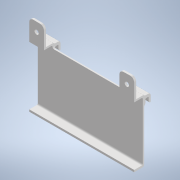
# Autodesk Inventor part: akkum_cup
Saved by Autodesk Inventor 2022 (Build 260153000, 153)
## iProperties
Created: 2024-11-13
Part Number: akkum_cup
Material: Типовые
Document SubType Name: Modeling
Designer: Andrey
Density: 1 g/cm^3
Appearance: По умолчанию
Author: Andrey
Autodesk Inventor part; units mm, degrees
ref_plane "YZ Plane" through (0, 0, 0) normal (1, 0, 0) x (0, 1, 0)
sketch "Эскиз1" plane through (0, 0, 0) normal (0, 0, 1) x (1, 0, 0)
  line L0 (39.5, 4.130031) -> (39.5, 47.075)
  line L1 (17.068713, 47.075) -> (39.5, 47.075)
  line L2 (17.068713, 47.075) -> (17.068713, 32.075)
  line L3 (17.068713, 32.075) -> (19.451364, 32.075)
  line L4 (19.451364, 32.075) -> (19.451364, 22.075)
  line L5 (19.451364, 22.075) -> (17.068713, 22.075)
  line L6 (17.068713, 22.075) -> (17.068713, 21.075)
  line L7 (17.068713, 21.075) -> (-5.922093, 21.075)
  line L8 (-5.922093, 21.075) -> (-5.922093, 47.075)
  line L9 (-39.5, 47.075) -> (-5.922093, 47.075)
  line L10 (-39.5, 47.075) -> (-39.5, 4.130031)
  line L11 (-39.5, 4.130031) -> (-43.5, 4.130031)
  line L12 (-43.5, -51.925) -> (-43.5, 4.130031)
  line L13 (43.5, -51.925) -> (-43.5, -51.925)
  line L14 (43.5, 4.130031) -> (43.5, -51.925)
  line L15 (43.5, 4.130031) -> (39.5, 4.130031)
  line L16 (-40, 47.075) -> (40, 47.075)
  line L17 (40, 47.075) -> (40, 7.075)
  line L18 (40, 7.075) -> (-40, 7.075)
  line L19 (-40, 7.075) -> (-40, 47.075)
  line L20 (39.5, -51.925) -> (-39.5, -51.925)
  line L21 (-39.5, -51.925) -> (-39.5, 106.075)
  line L22 (-39.5, 106.075) -> (39.5, 106.075)
  line L23 (39.5, 106.075) -> (39.5, -51.925)
  line L24 (-40, 50.145438) -> (-43.5, 50.145438)
  line L25 (-43.5, 50.145438) -> (-43.5, 87.075)
  line L26 (-43.5, 87.075) -> (-62.794737, 87.075)
  line L27 (-62.794737, 87.075) -> (-62.794737, -32.925)
  line L28 (-62.794737, -32.925) -> (-43.5, -32.925)
  line L29 (-43.5, -32.925) -> (-43.5, 5.130031)
  line L30 (-43.5, 5.130031) -> (43.5, 5.130031)
  line L31 (43.5, 5.130031) -> (43.5, -32.925)
  line L32 (43.5, -32.925) -> (62.794737, -32.925)
  line L33 (62.794737, -32.925) -> (62.794737, 87.075)
  line L34 (62.794737, 87.075) -> (43.5, 87.075)
  line L35 (43.5, 87.075) -> (43.5, 50.145438)
  line L36 (43.5, 50.145438) -> (40, 50.145438)
  line L37 (40, 50.145438) -> (40, 49.145438)
  line L38 (40, 49.145438) -> (27.613813, 49.145438)
  line L39 (27.613813, 49.145438) -> (27.613813, 50.271275)
  line L40 (27.613813, 50.271275) -> (10.238021, 50.271275)
  line L41 (10.238021, 50.271275) -> (10.238021, 49.145438)
  line L42 (10.238021, 49.145438) -> (5, 49.145438)
  line L43 (5, 49.145438) -> (5, 52.145438)
  line L44 (5, 52.145438) -> (-5, 52.145438)
  line L45 (-5, 52.145438) -> (-5, 49.145438)
  line L46 (-5, 49.145438) -> (-10.238021, 49.145438)
  line L47 (-10.238021, 49.145438) -> (-10.238021, 50.271275)
  line L48 (-10.238021, 50.271275) -> (-27.613813, 50.271275)
  line L49 (-27.613813, 50.271275) -> (-27.613813, 49.145438)
  line L50 (-27.613813, 49.145438) -> (-40, 49.145438)
  line L51 (-40, 49.145438) -> (-40, 50.145438)
  line L52 (-40.5, -9.071748) -> (-40.5, -29.675)
  line L53 (-40.5, -29.675) -> (-25.5, -29.675)
  line L54 (-25.5, -29.675) -> (-25.5, -9.071748)
  line L55 (-25.5, -9.071748) -> (-40.5, -9.071748)
  circle A0 centre (-35.935126, 58.395438) radius 2.1
  circle A1 centre (-23.0037, 78.773688) radius 2.1
  circle A2 centre (23.0037, 78.773688) radius 2.1
  circle A3 centre (35.954001, 58.395438) radius 2.1
  line L56 (-5, 87.075) -> (5, 87.075)
  line L57 (5, 87.075) -> (5, 106.075)
  line L58 (5, 106.075) -> (52.763624, 106.075)
  spline S0 degree 4 poles (64.11012, 98.855268) (61.979597, 102.169879) (57.930304, 105.392192) (55.716138, 106.075) (52.763624, 106.075) knots 0 0 0 0 0 1 1 1 1 1
  spline S1 degree 2 poles (66.794737, 82.075) (67.198697, 94.050143) (64.11012, 98.855268) knots 0 0 0 0.59571899 0.59571899 0.59571899
  line L59 (66.794737, -27.925) -> (66.794737, 82.075)
  spline S2 degree 2 poles (66.794737, -27.925) (67.198697, -39.900143) (64.11012, -44.705268) knots 0 0 0 0.59571899 0.59571899 0.59571899
  spline S3 degree 4 poles (64.11012, -44.705268) (64.099074, -44.722454) (64.087976, -44.739637) (64.076827, -44.756817) (64.065627, -44.773995) knots 0 0 0 0 0 1 1 1 1 1
  spline S4 degree 4 poles (63.235072, -45.91909) (63.456659, -45.667632) (63.669141, -45.393003) (63.87219, -45.095007) (64.065627, -44.773995) knots 0 0 0 0 0 1 1 1 1 1
  spline S5 degree 4 poles (63.235072, -45.91909) (60.901345, -48.850089) (57.514512, -51.362629) (55.443125, -51.925) (52.763624, -51.925) knots 0.09246802 0.09246802 0.09246802 0.09246802 0.09246802 1 1 1 1 1
  line L60 (6, -51.925) -> (52.763624, -51.925)
  line L61 (6, -51.925) -> (6, -36.071748)
  arc A4 (6, -36.071748) -> (5, -35.071748) centre (5, -36.071748) ccw
  line L62 (5, -35.071748) -> (-5, -35.071748)
  arc A5 (-5, -35.071748) -> (-6, -36.071748) centre (-5, -36.071748) ccw
  line L63 (-6, -36.071748) -> (-6, -51.925)
  line L64 (-52.763624, -51.925) -> (-6, -51.925)
  spline S6 degree 4 poles (-64.11012, -44.705268) (-61.979597, -48.019879) (-57.930304, -51.242192) (-55.716138, -51.925) (-52.763624, -51.925) knots 0 0 0 0 0 1 1 1 1 1
  spline S7 degree 2 poles (-66.794737, -27.925) (-67.198697, -39.900143) (-64.11012, -44.705268) knots 0 0 0 0.59571899 0.59571899 0.59571899
  line L65 (-66.794737, 82.075) -> (-66.794737, -27.925)
  spline S8 degree 2 poles (-64.11012, 98.855268) (-67.198697, 94.050143) (-66.794737, 82.075) knots -0.59571899 -0.59571899 -0.59571899 0 0 0
  spline S9 degree 4 poles (-64.11012, 98.855268) (-61.979597, 102.169879) (-57.930304, 105.392192) (-55.716138, 106.075) (-52.763624, 106.075) knots 0 0 0 0 0 1 1 1 1 1
  line L66 (-52.763624, 106.075) -> (-5, 106.075)
  line L67 (-5, 106.075) -> (-5, 87.075)
  line L68 (-33.1, -33.525) -> (-40.1, -33.525)
  line L69 (-40.1, -33.525) -> (-40.1, -47.625)
  line L70 (-40.1, -47.625) -> (-33.1, -47.625)
  line L71 (-33.1, -47.625) -> (-33.1, -33.525)
  line L72 (40.1, -33.675) -> (33.1, -33.675)
  line L73 (33.1, -33.675) -> (33.1, -47.625)
  line L74 (33.1, -47.625) -> (40.1, -47.625)
  line L75 (40.1, -47.625) -> (40.1, -33.675)
  line L76 (3.8, 77.044784) -> (-15.7, 77.044784)
  arc A6 (-15.7, 77.044784) -> (-18.7, 74.044784) centre (-15.7, 74.044784) ccw
  line L77 (-18.7, 74.044784) -> (-18.7, 60.781085)
  arc A7 (-18.7, 60.781085) -> (-15.7, 57.781085) centre (-15.7, 60.781085) ccw
  line L78 (-15.7, 57.781085) -> (3.8, 57.781085)
  arc A8 (3.8, 57.781085) -> (6.8, 60.781085) centre (3.8, 60.781085) ccw
  line L79 (6.8, 60.781085) -> (6.8, 74.044784)
  arc A9 (6.8, 74.044784) -> (3.8, 77.044784) centre (3.8, 74.044784) ccw
  line L80 (39.5, 49.145438) -> (-39.5, 49.145438)
  line L81 (-37.533703, 49.795438) -> (-66.794737, 49.795438)
  line L82 (-66.794737, 49.795438) -> (66.794737, 49.795438)
  line L83 (66.794737, 3.630031) -> (-65.776453, 3.630031)
  line L84 (-40, 50.145438) -> (-43.5, 50.145438)
  line L85 (-43.5, 50.145438) -> (-43.5, 87.075)
  line L86 (-43.5, 87.075) -> (-62.794737, 87.075)
  line L87 (-62.794737, 87.075) -> (-62.794737, -32.925)
  line L88 (-62.794737, -32.925) -> (-43.5, -32.925)
  line L89 (-43.5, -32.925) -> (-43.5, 5.130031)
  line L90 (-43.5, 5.130031) -> (43.5, 5.130031)
  line L91 (43.5, 5.130031) -> (43.5, -32.925)
  line L92 (43.5, -32.925) -> (62.794737, -32.925)
  line L93 (62.794737, -32.925) -> (62.794737, 87.075)
  line L94 (62.794737, 87.075) -> (43.5, 87.075)
  line L95 (43.5, 87.075) -> (43.5, 50.145438)
  line L96 (43.5, 50.145438) -> (40, 50.145438)
  line L97 (40, 50.145438) -> (40, 49.145438)
  line L98 (40, 49.145438) -> (27.613813, 49.145438)
  line L99 (27.613813, 49.145438) -> (27.613813, 50.271275)
  line L100 (27.613813, 50.271275) -> (10.238021, 50.271275)
  line L101 (10.238021, 50.271275) -> (10.238021, 49.145438)
  line L102 (10.238021, 49.145438) -> (5, 49.145438)
  line L103 (5, 49.145438) -> (5, 52.145438)
  line L104 (5, 52.145438) -> (-5, 52.145438)
  line L105 (-5, 52.145438) -> (-5, 49.145438)
  line L106 (-5, 49.145438) -> (-10.238021, 49.145438)
  line L107 (-10.238021, 49.145438) -> (-10.238021, 50.271275)
  line L108 (-10.238021, 50.271275) -> (-27.613813, 50.271275)
  line L109 (-27.613813, 50.271275) -> (-27.613813, 49.145438)
  line L110 (-27.613813, 49.145438) -> (-40, 49.145438)
  line L111 (-40, 49.145438) -> (-40, 50.145438)
  line L112 (-40.5, -9.071748) -> (-40.5, -29.675)
  line L113 (-40.5, -29.675) -> (-25.5, -29.675)
  line L114 (-25.5, -29.675) -> (-25.5, -9.071748)
  line L115 (-25.5, -9.071748) -> (-40.5, -9.071748)
  circle A10 centre (-35.935126, 58.395438) radius 2.1
  circle A11 centre (-23.0037, 78.773688) radius 2.1
  circle A12 centre (23.0037, 78.773688) radius 2.1
  circle A13 centre (35.954001, 58.395438) radius 2.1
  line L116 (-5, 87.075) -> (5, 87.075)
  line L117 (5, 87.075) -> (5, 106.075)
  line L118 (5, 106.075) -> (52.763624, 106.075)
  spline S10 degree 4 poles (64.11012, 98.855268) (61.979597, 102.169879) (57.930304, 105.392192) (55.716138, 106.075) (52.763624, 106.075) knots 0 0 0 0 0 1 1 1 1 1
  spline S11 degree 2 poles (66.794737, 82.075) (67.198697, 94.050143) (64.11012, 98.855268) knots 0 0 0 0.59571899 0.59571899 0.59571899
  line L119 (66.794737, -27.925) -> (66.794737, 82.075)
  spline S12 degree 2 poles (66.794737, -27.925) (67.198697, -39.900143) (64.11012, -44.705268) knots 0 0 0 0.59571899 0.59571899 0.59571899
  spline S13 degree 4 poles (64.11012, -44.705268) (64.099074, -44.722454) (64.087976, -44.739637) (64.076827, -44.756817) (64.065627, -44.773995) knots 0 0 0 0 0 1 1 1 1 1
  spline S14 degree 4 poles (63.235072, -45.91909) (63.456659, -45.667632) (63.669141, -45.393003) (63.87219, -45.095007) (64.065627, -44.773995) knots 0 0 0 0 0 1 1 1 1 1
  spline S15 degree 4 poles (63.235072, -45.91909) (60.901345, -48.850089) (57.514512, -51.362629) (55.443125, -51.925) (52.763624, -51.925) knots 0.09246802 0.09246802 0.09246802 0.09246802 0.09246802 1 1 1 1 1
  line L120 (6, -51.925) -> (52.763624, -51.925)
  line L121 (6, -51.925) -> (6, -36.071748)
  arc A14 (6, -36.071748) -> (5, -35.071748) centre (5, -36.071748) ccw
  line L122 (5, -35.071748) -> (-5, -35.071748)
  arc A15 (-5, -35.071748) -> (-6, -36.071748) centre (-5, -36.071748) ccw
  line L123 (-6, -36.071748) -> (-6, -51.925)
  line L124 (-52.763624, -51.925) -> (-6, -51.925)
  spline S16 degree 4 poles (-64.11012, -44.705268) (-61.979597, -48.019879) (-57.930304, -51.242192) (-55.716138, -51.925) (-52.763624, -51.925) knots 0 0 0 0 0 1 1 1 1 1
  spline S17 degree 2 poles (-66.794737, -27.925) (-67.198697, -39.900143) (-64.11012, -44.705268) knots 0 0 0 0.59571899 0.59571899 0.59571899
  line L125 (-66.794737, 82.075) -> (-66.794737, -27.925)
  spline S18 degree 2 poles (-64.11012, 98.855268) (-67.198697, 94.050143) (-66.794737, 82.075) knots -0.59571899 -0.59571899 -0.59571899 0 0 0
  spline S19 degree 4 poles (-64.11012, 98.855268) (-61.979597, 102.169879) (-57.930304, 105.392192) (-55.716138, 106.075) (-52.763624, 106.075) knots 0 0 0 0 0 1 1 1 1 1
  line L126 (-52.763624, 106.075) -> (-5, 106.075)
  line L127 (-5, 106.075) -> (-5, 87.075)
  line L128 (-33.1, -33.525) -> (-40.1, -33.525)
  line L129 (-40.1, -33.525) -> (-40.1, -47.625)
  line L130 (-40.1, -47.625) -> (-33.1, -47.625)
  line L131 (-33.1, -47.625) -> (-33.1, -33.525)
  line L132 (40.1, -33.675) -> (33.1, -33.675)
  line L133 (33.1, -33.675) -> (33.1, -47.625)
  line L134 (33.1, -47.625) -> (40.1, -47.625)
  line L135 (40.1, -47.625) -> (40.1, -33.675)
  line L136 (3.8, 77.044784) -> (-15.7, 77.044784)
  arc A16 (-15.7, 77.044784) -> (-18.7, 74.044784) centre (-15.7, 74.044784) ccw
  line L137 (-18.7, 74.044784) -> (-18.7, 60.781085)
  arc A17 (-18.7, 60.781085) -> (-15.7, 57.781085) centre (-15.7, 60.781085) ccw
  line L138 (-15.7, 57.781085) -> (3.8, 57.781085)
  arc A18 (3.8, 57.781085) -> (6.8, 60.781085) centre (3.8, 60.781085) ccw
  line L139 (6.8, 60.781085) -> (6.8, 74.044784)
  arc A19 (6.8, 74.044784) -> (3.8, 77.044784) centre (3.8, 74.044784) ccw
  line L140 (27.613813, 49.145438) -> (27.613813, 47.075)
  line L141 (-27.613813, 49.145438) -> (-27.613813, 47.075)
  line L142 (-28.408002, 50.795438) -> (-28.408002, 49.795438)
  line L143 (28.408002, 49.795438) -> (28.408002, 50.795438)
  line L144 (28.408002, 50.795438) -> (43.5, 50.795438)
  line L145 (-43.5, 50.795438) -> (-28.408002, 50.795438)
  line L146 (43.5, 50.795438) -> (-43.5, 50.795438)
  line L147 (43.5, 50.495438) -> (-43.5, 50.495438)
  line L148 (-28.408002, 50.495438) -> (-28.408002, 47.075)
  line L149 (28.408002, 50.495438) -> (28.408002, 47.075)
  point P0 (0, 0)
  point P1 (39.5, 49.795438)
  point P2 (27.613813, 49.795438)
  point P3 (-27.613813, 49.795438)
  point P4 (-39.5, 49.795438)
  point P5 (-39.5, 3.630031)
  point P6 (39.5, 3.630031)
  point P7 (-39.5, 50.495438)
  point P8 (39.5, 50.495438)
  dimension "d0" = 1.5
  dimension "d7" = 0.3
  constraints: 32 end point, 13 point on line, 7 perpendicular, 4 collinear, 4 parallel, 3 horizontal, 2 vertical, 6 other
  measures "d0" distance between parallel lines of L30 L83
  measures "d7" distance between parallel lines of L146 L147
extrude "Выдавливание1" add sketch "Эскиз1" along normal blind 2 contours L23 L83 L21 L10 L30 L0 | L30 L10 L18 L0 | L18 L10 L9 L8 L7 L6 L5 L4 L3 L2 L1 L0 | L1 L149 L38 L23 | L38 L149 L82 L23 | L21 L50 L148 L9 | L82 L143 L147 L23 | L21 L81 L82 L148 L50 | L2 L3 L4 L5 L6 L7 L8 L16 | L21 L147 L142 L82 L81
sketch "Эскиз2" plane through (-39.5, 3.630031, 0) normal (-1, 0, 0) x (0, 0, 1)
  line L0 (0, 0) -> (2, 0)
  line L1 (1, 0) -> (1, 46.165408)
  line L2 (0, 46.165408) -> (2, 46.165408)
  line L3 (0, 46.865408) -> (0, 0)
  line L4 (0, 0) -> (2, 0)
  line L5 (2, 46.865408) -> (2, 0)
  line L6 (0, 46.865408) -> (2, 46.865408)
  line L7 (0, 46.865408) -> (2, 46.865408)
  line L8 (1, 46.865408) -> (1, 0)
  point P0 (0, -3.630031)
  point P1 (0, 0)
  constraints: 4 end point, 3 midpoint, 1 collinear
extrude "Выдавливание2" cut sketch "Эскиз2" against normal up to surface (79 mm away) contours L3 L2 L1 L0 | L3 L6 L8 L2
ref_plane "РабПлоскость1" through (-67.197727, -51.925, 8.5) normal (0, 0, -1) x (0, 1, 0)
sketch "Эскиз3" plane through (0, 0, 2) normal (0, 0, 1) x (1, 0, 0)
  line L0 (39.5, 3.630031) -> (39.5, 50.495438)
  line L1 (-39.5, 50.495438) -> (-39.5, 3.630031)
  line L2 (-39.5, 3.630031) -> (39.5, 3.630031)
  line L3 (-27.613813, 49.795438) -> (-39.5, 49.795438)
  line L4 (39.5, 3.630031) -> (39.5, 50.495438)
  line L5 (-39.5, 49.795438) -> (39.5, 49.795438)
  line L6 (39.5, 49.795438) -> (39.5, 49.145438)
  line L7 (39.5, 49.145438) -> (-39.5, 49.145438)
  line L8 (-39.5, 49.145438) -> (-39.5, 49.795438)
  line L9 (-40, 50.145438) -> (-43.5, 50.145438)
  line L10 (-43.5, 50.145438) -> (-43.5, 87.075)
  line L11 (-43.5, 87.075) -> (-62.794737, 87.075)
  line L12 (-62.794737, 87.075) -> (-62.794737, -32.925)
  line L13 (-62.794737, -32.925) -> (-43.5, -32.925)
  line L14 (-43.5, -32.925) -> (-43.5, 5.130031)
  line L15 (-43.5, 5.130031) -> (43.5, 5.130031)
  line L16 (43.5, 5.130031) -> (43.5, -32.925)
  line L17 (43.5, -32.925) -> (62.794737, -32.925)
  line L18 (62.794737, -32.925) -> (62.794737, 87.075)
  line L19 (62.794737, 87.075) -> (43.5, 87.075)
  line L20 (43.5, 87.075) -> (43.5, 50.145438)
  line L21 (43.5, 50.145438) -> (40, 50.145438)
  line L22 (40, 50.145438) -> (40, 49.145438)
  line L23 (40, 49.145438) -> (27.613813, 49.145438)
  line L24 (27.613813, 49.145438) -> (27.613813, 50.271275)
  line L25 (27.613813, 50.271275) -> (10.238021, 50.271275)
  line L26 (10.238021, 50.271275) -> (10.238021, 49.145438)
  line L27 (10.238021, 49.145438) -> (5, 49.145438)
  line L28 (5, 49.145438) -> (5, 52.145438)
  line L29 (5, 52.145438) -> (-5, 52.145438)
  line L30 (-5, 52.145438) -> (-5, 49.145438)
  line L31 (-5, 49.145438) -> (-10.238021, 49.145438)
  line L32 (-10.238021, 49.145438) -> (-10.238021, 50.271275)
  line L33 (-10.238021, 50.271275) -> (-27.613813, 50.271275)
  line L34 (-27.613813, 50.271275) -> (-27.613813, 49.145438)
  line L35 (-27.613813, 49.145438) -> (-40, 49.145438)
  line L36 (-40, 49.145438) -> (-40, 50.145438)
  line L37 (-40.5, -9.071748) -> (-40.5, -29.675)
  line L38 (-40.5, -29.675) -> (-25.5, -29.675)
  line L39 (-25.5, -29.675) -> (-25.5, -9.071748)
  line L40 (-25.5, -9.071748) -> (-40.5, -9.071748)
  circle A0 centre (-35.935126, 58.395438) radius 2.1
  circle A1 centre (-23.0037, 78.773688) radius 2.1
  circle A2 centre (23.0037, 78.773688) radius 2.1
  circle A3 centre (35.954001, 58.395438) radius 2.1
  line L41 (-5, 87.075) -> (5, 87.075)
  line L42 (5, 87.075) -> (5, 106.075)
  line L43 (5, 106.075) -> (52.763624, 106.075)
  spline S0 degree 4 poles (64.11012, 98.855268) (61.979597, 102.169879) (57.930304, 105.392192) (55.716138, 106.075) (52.763624, 106.075) knots 0 0 0 0 0 1 1 1 1 1
  spline S1 degree 2 poles (66.794737, 82.075) (67.198697, 94.050143) (64.11012, 98.855268) knots 0 0 0 0.59571899 0.59571899 0.59571899
  line L44 (66.794737, -27.925) -> (66.794737, 82.075)
  spline S2 degree 2 poles (66.794737, -27.925) (67.198697, -39.900143) (64.11012, -44.705268) knots 0 0 0 0.59571899 0.59571899 0.59571899
  spline S3 degree 4 poles (64.11012, -44.705268) (64.099074, -44.722454) (64.087976, -44.739637) (64.076827, -44.756817) (64.065627, -44.773995) knots 0 0 0 0 0 1 1 1 1 1
  spline S4 degree 4 poles (63.235072, -45.91909) (63.456659, -45.667632) (63.669141, -45.393003) (63.87219, -45.095007) (64.065627, -44.773995) knots 0 0 0 0 0 1 1 1 1 1
  spline S5 degree 4 poles (63.235072, -45.91909) (60.901345, -48.850089) (57.514512, -51.362629) (55.443125, -51.925) (52.763624, -51.925) knots 0.09246802 0.09246802 0.09246802 0.09246802 0.09246802 1 1 1 1 1
  line L45 (6, -51.925) -> (52.763624, -51.925)
  line L46 (6, -51.925) -> (6, -36.071748)
  arc A4 (6, -36.071748) -> (5, -35.071748) centre (5, -36.071748) ccw
  line L47 (5, -35.071748) -> (-5, -35.071748)
  arc A5 (-5, -35.071748) -> (-6, -36.071748) centre (-5, -36.071748) ccw
  line L48 (-6, -36.071748) -> (-6, -51.925)
  line L49 (-52.763624, -51.925) -> (-6, -51.925)
  spline S6 degree 4 poles (-64.11012, -44.705268) (-61.979597, -48.019879) (-57.930304, -51.242192) (-55.716138, -51.925) (-52.763624, -51.925) knots 0 0 0 0 0 1 1 1 1 1
  spline S7 degree 2 poles (-66.794737, -27.925) (-67.198697, -39.900143) (-64.11012, -44.705268) knots 0 0 0 0.59571899 0.59571899 0.59571899
  line L50 (-66.794737, 82.075) -> (-66.794737, -27.925)
  spline S8 degree 2 poles (-64.11012, 98.855268) (-67.198697, 94.050143) (-66.794737, 82.075) knots -0.59571899 -0.59571899 -0.59571899 0 0 0
  spline S9 degree 4 poles (-64.11012, 98.855268) (-61.979597, 102.169879) (-57.930304, 105.392192) (-55.716138, 106.075) (-52.763624, 106.075) knots 0 0 0 0 0 1 1 1 1 1
  line L51 (-52.763624, 106.075) -> (-5, 106.075)
  line L52 (-5, 106.075) -> (-5, 87.075)
  line L53 (-33.1, -33.525) -> (-40.1, -33.525)
  line L54 (-40.1, -33.525) -> (-40.1, -47.625)
  line L55 (-40.1, -47.625) -> (-33.1, -47.625)
  line L56 (-33.1, -47.625) -> (-33.1, -33.525)
  line L57 (40.1, -33.675) -> (33.1, -33.675)
  line L58 (33.1, -33.675) -> (33.1, -47.625)
  line L59 (33.1, -47.625) -> (40.1, -47.625)
  line L60 (40.1, -47.625) -> (40.1, -33.675)
  line L61 (3.8, 77.044784) -> (-15.7, 77.044784)
  arc A6 (-15.7, 77.044784) -> (-18.7, 74.044784) centre (-15.7, 74.044784) ccw
  line L62 (-18.7, 74.044784) -> (-18.7, 60.781085)
  arc A7 (-18.7, 60.781085) -> (-15.7, 57.781085) centre (-15.7, 60.781085) ccw
  line L63 (-15.7, 57.781085) -> (3.8, 57.781085)
  arc A8 (3.8, 57.781085) -> (6.8, 60.781085) centre (3.8, 60.781085) ccw
  line L64 (6.8, 60.781085) -> (6.8, 74.044784)
  arc A9 (6.8, 74.044784) -> (3.8, 77.044784) centre (3.8, 74.044784) ccw
  line L65 (28.408002, 47.075) -> (-28.408002, 47.075)
  line L66 (-28.408002, 47.075) -> (-28.408002, 50.495438)
  line L67 (-28.408002, 50.495438) -> (-39.5, 50.495438)
  line L68 (39.5, 50.495438) -> (28.408002, 50.495438)
  line L69 (28.408002, 50.495438) -> (28.408002, 47.075)
  point P0 (0, 0)
  point P1 (39.5, 49.795438)
  point P2 (27.613813, 49.795438)
  point P3 (-39.5, 49.145438)
  point P4 (39.5, 5.130031)
  point P5 (-39.5, 5.130031)
  point P6 (-28.408002, 49.145438)
  point P7 (28.408002, 49.145438)
  constraints: 8 end point, 2 parallel, 1 collinear, 1 horizontal, 1 perpendicular, 1 point on line
extrude "Выдавливание3" add sketch "Эскиз3" along normal up to surface (6.5 mm away) contours L7 L69 L5 L0 | L5 L69 L68 L0 | L0 L2 L1 L15 | L1 L3 L66 L7 | L1 L67 L66 L3
fillet "Сопряжение1" radius 1 6 edges at (-33.954, 49.1454, 2) (-33.954, 50.4954, 1) (33.954, 49.1454, 2) (33.954, 50.4954, 1) (0, 3.63, 1) (0, 5.13, 2)
sketch "Эскиз4" plane through (0, 0, 8.5) normal (0, 0, 1) x (1, 0, 0)
  line L0 (28.408002, 50.495438) -> (28.408002, 49.145438)
  line L1 (39.5, 50.495438) -> (28.408002, 50.495438)
  line L2 (40, 49.145438) -> (27.613813, 49.145438)
  line L3 (39.5, 49.145438) -> (39.5, 50.495438)
  line L4 (-28.408002, 50.495438) -> (-39.5, 50.495438)
  line L5 (-28.408002, 49.145438) -> (-28.408002, 50.495438)
  line L6 (-27.613813, 49.145438) -> (-40, 49.145438)
  line L7 (-39.5, 50.495438) -> (-39.5, 49.145438)
  line L8 (-39.5, 5.130031) -> (39.5, 5.130031)
  line L9 (39.5, 5.130031) -> (-39.5, 5.130031)
  line L10 (-39.5, 3.630031) -> (39.5, 3.630031)
  line L11 (-39.5, 5.130031) -> (-39.5, 3.630031)
  line L12 (39.5, 3.630031) -> (39.5, 5.130031)
  line L13 (-28.108002, 50.121275) -> (-10.238021, 50.121275)
  ellipse E0 centre (0, 75.849578) end of major axis (0, 36.378218) minor radius 13.5 (-11.262267, 54.085128) -> (-10.238021, 50.121275) ccw
  line L14 (-11.262267, 54.085128) -> (11.262267, 54.085128)
  ellipse E1 centre (0, 75.849578) end of major axis (0, 36.378218) minor radius 13.5 (10.238021, 50.121275) -> (11.262267, 54.085128) ccw
  line L15 (10.238021, 50.121275) -> (28.108002, 50.121275)
  line L16 (28.408002, 65.262392) -> (28.408002, 66.695438)
  line L17 (28.408002, 66.695438) -> (5.950174, 66.695438)
  ellipse E2 centre (1.3, 74.130116) end of major axis (1.3, 58.633952) minor radius 5.3 (1.3, 58.633952) -> (5.950174, 66.695438) ccw
  line L18 (-13.2, 58.633952) -> (1.3, 58.633952)
  ellipse E3 centre (-13.2, 74.130116) end of major axis (-13.2, 58.633952) minor radius 5.3 (-17.850174, 66.695438) -> (-13.2, 58.633952) ccw
  line L19 (-17.850174, 66.695438) -> (-28.408002, 66.695438)
  line L20 (-28.408002, 66.695438) -> (-28.408002, 65.262392)
  line L21 (39.5, 49.145438) -> (28.408002, 49.145438)
  line L22 (28.408002, 49.145438) -> (28.408002, 64.962323)
  line L23 (28.408002, 64.962323) -> (39.5, 65.200767)
  line L24 (39.5, 65.200767) -> (39.5, 49.145438)
  line L25 (-28.408002, 50.495438) -> (-39.5, 50.495438)
  line L26 (-39.5, 50.495438) -> (-39.5, 65.200767)
  line L27 (-39.5, 65.200767) -> (-28.408002, 64.962323)
  line L28 (-28.408002, 64.962323) -> (-28.408002, 50.495438)
  line L29 (39.5, 5.130031) -> (-32.5, 5.130031)
  line L30 (-32.5, 5.130031) -> (-32.5, -4.369969)
  line L31 (-32.5, -4.369969) -> (32.5, -4.369969)
  line L32 (-28.408002, 65.262392) -> (-28.108002, 65.255943)
  line L33 (-28.108002, 65.255943) -> (-28.108002, 50.121275)
  line L34 (28.108002, 50.121275) -> (28.108002, 65.255943)
  line L35 (28.108002, 65.255943) -> (28.408002, 65.262392)
  circle A0 centre (-33.954001, 58.245438) radius 2.1
  circle A1 centre (33.954001, 58.245438) radius 2.1
  line L36 (-43.469718, 66.695438) -> (-28.408002, 66.695438)
  line L37 (43.469718, 66.695438) -> (28.408002, 66.695438)
  circle A2 centre (-33.954001, 58.245438) radius 1.6
  circle A3 centre (33.954001, 58.245438) radius 1.6
  line L38 (-32.5, -4.369969) -> (-28.408002, -4.369969)
  line L39 (-28.408002, -4.369969) -> (-28.408002, 50.495438)
  line L40 (-28.408002, 50.495438) -> (-32.5, 50.495438)
  line L41 (-32.5, 50.495438) -> (-32.5, -4.369969)
  line L42 (32.5, -4.369969) -> (28.408002, -4.369969)
  line L43 (28.408002, -4.369969) -> (28.408002, 50.495438)
  line L44 (28.408002, 50.495438) -> (32.5, 50.495438)
  line L45 (32.5, 50.495438) -> (32.5, -4.369969)
  line L46 (-40, 50.145438) -> (-43.5, 50.145438)
  line L47 (-43.5, 50.145438) -> (-43.5, 87.075)
  line L48 (-43.5, 87.075) -> (-62.794737, 87.075)
  line L49 (-62.794737, 87.075) -> (-62.794737, -32.925)
  line L50 (-62.794737, -32.925) -> (-43.5, -32.925)
  line L51 (-43.5, -32.925) -> (-43.5, 5.130031)
  line L52 (-43.5, 5.130031) -> (43.5, 5.130031)
  line L53 (43.5, 5.130031) -> (43.5, -32.925)
  line L54 (43.5, -32.925) -> (62.794737, -32.925)
  line L55 (62.794737, -32.925) -> (62.794737, 87.075)
  line L56 (62.794737, 87.075) -> (43.5, 87.075)
  line L57 (43.5, 87.075) -> (43.5, 50.145438)
  line L58 (43.5, 50.145438) -> (40, 50.145438)
  line L59 (40, 50.145438) -> (40, 49.145438)
  line L60 (40, 49.145438) -> (27.613813, 49.145438)
  line L61 (27.613813, 49.145438) -> (27.613813, 50.271275)
  line L62 (27.613813, 50.271275) -> (10.238021, 50.271275)
  line L63 (10.238021, 50.271275) -> (10.238021, 49.145438)
  line L64 (10.238021, 49.145438) -> (5, 49.145438)
  line L65 (5, 49.145438) -> (5, 52.145438)
  line L66 (5, 52.145438) -> (-5, 52.145438)
  line L67 (-5, 52.145438) -> (-5, 49.145438)
  line L68 (-5, 49.145438) -> (-10.238021, 49.145438)
  line L69 (-10.238021, 49.145438) -> (-10.238021, 50.271275)
  line L70 (-10.238021, 50.271275) -> (-27.613813, 50.271275)
  line L71 (-27.613813, 50.271275) -> (-27.613813, 49.145438)
  line L72 (-27.613813, 49.145438) -> (-40, 49.145438)
  line L73 (-40, 49.145438) -> (-40, 50.145438)
  line L74 (-40.5, -9.071748) -> (-40.5, -29.675)
  line L75 (-40.5, -29.675) -> (-25.5, -29.675)
  line L76 (-25.5, -29.675) -> (-25.5, -9.071748)
  line L77 (-25.5, -9.071748) -> (-40.5, -9.071748)
  circle A4 centre (-33.954001, 58.245438) radius 1.5
  circle A5 centre (-23.004634, 78.74639) radius 1.5
  circle A6 centre (23.004634, 78.74639) radius 1.5
  circle A7 centre (33.954001, 58.245438) radius 1.5
  line L78 (-5, 87.075) -> (5, 87.075)
  line L79 (5, 87.075) -> (5, 106.075)
  line L80 (5, 106.075) -> (52.763624, 106.075)
  spline S0 degree 4 poles (64.109599, 98.855027) (61.979127, 102.16956) (57.930153, 105.39205) (55.716058, 106.075) (52.763624, 106.075) knots 0 0 0 0 0 1 1 1 1 1
  spline S1 degree 2 poles (66.794737, 82.075) (67.198212, 94.049847) (64.109599, 98.855027) knots 0 0 0 0.59573075 0.59573075 0.59573075
  line L81 (66.794737, -27.925) -> (66.794737, 82.075)
  spline S2 degree 2 poles (66.794737, -27.925) (67.198212, -39.899847) (64.109599, -44.705027) knots 0 0 0 0.59573075 0.59573075 0.59573075
  spline S3 degree 4 poles (64.109599, -44.705027) (64.100707, -44.718862) (64.091781, -44.732695) (64.082822, -44.746527) (64.07383, -44.760356) knots 0 0 0 0 0 1 1 1 1 1
  spline S4 degree 4 poles (63.227931, -45.927181) (63.453878, -45.6716) (63.670381, -45.391979) (63.877095, -45.088106) (64.07383, -44.760356) knots 0 0 0 0 0 1 1 1 1 1
  spline S5 degree 4 poles (63.227931, -45.927181) (60.893724, -48.855183) (57.511423, -51.363314) (55.441144, -51.925) (52.763624, -51.925) knots 0.09311431 0.09311431 0.09311431 0.09311431 0.09311431 1 1 1 1 1
  line L82 (6, -51.925) -> (52.763624, -51.925)
  line L83 (6, -51.925) -> (6, -36.071748)
  arc A8 (6, -36.071748) -> (5, -35.071748) centre (5, -36.071748) ccw
  line L84 (5, -35.071748) -> (-5, -35.071748)
  arc A9 (-5, -35.071748) -> (-6, -36.071748) centre (-5, -36.071748) ccw
  line L85 (-6, -36.071748) -> (-6, -51.925)
  line L86 (-52.763624, -51.925) -> (-6, -51.925)
  spline S6 degree 4 poles (-64.109599, -44.705027) (-61.979127, -48.01956) (-57.930153, -51.24205) (-55.716058, -51.925) (-52.763624, -51.925) knots 0 0 0 0 0 1 1 1 1 1
  spline S7 degree 2 poles (-66.794737, -27.925) (-67.198212, -39.899847) (-64.109599, -44.705027) knots 0 0 0 0.59573075 0.59573075 0.59573075
  line L87 (-66.794737, 82.075) -> (-66.794737, -27.925)
  spline S8 degree 2 poles (-64.109599, 98.855027) (-67.198212, 94.049847) (-66.794737, 82.075) knots -0.59573075 -0.59573075 -0.59573075 0 0 0
  spline S9 degree 4 poles (-64.109599, 98.855027) (-61.979127, 102.16956) (-57.930153, 105.39205) (-55.716058, 106.075) (-52.763624, 106.075) knots 0 0 0 0 0 1 1 1 1 1
  line L88 (-52.763624, 106.075) -> (-5, 106.075)
  line L89 (-5, 106.075) -> (-5, 87.075)
  line L90 (-33.1, -33.525) -> (-40.1, -33.525)
  line L91 (-40.1, -33.525) -> (-40.1, -47.625)
  line L92 (-40.1, -47.625) -> (-33.1, -47.625)
  line L93 (-33.1, -47.625) -> (-33.1, -33.525)
  line L94 (40.1, -33.675) -> (33.1, -33.675)
  line L95 (33.1, -33.675) -> (33.1, -47.625)
  line L96 (33.1, -47.625) -> (40.1, -47.625)
  line L97 (40.1, -47.625) -> (40.1, -33.675)
  line L98 (3.8, 77.044784) -> (-15.7, 77.044784)
  arc A10 (-15.7, 77.044784) -> (-18.7, 74.044784) centre (-15.7, 74.044784) ccw
  line L99 (-18.7, 74.044784) -> (-18.7, 60.781085)
  arc A11 (-18.7, 60.781085) -> (-15.7, 57.781085) centre (-15.7, 60.781085) ccw
  line L100 (-15.7, 57.781085) -> (3.8, 57.781085)
  arc A12 (3.8, 57.781085) -> (6.8, 60.781085) centre (3.8, 60.781085) ccw
  line L101 (6.8, 60.781085) -> (6.8, 74.044784)
  arc A13 (6.8, 74.044784) -> (3.8, 77.044784) centre (3.8, 74.044784) ccw
  line L102 (-32.5, -0.369969) -> (32.5, -0.369969)
  line L103 (24.5, -4.369969) -> (24.5, 3.630031)
  line L104 (-24.5, -4.369969) -> (-24.5, 3.630031)
  circle A14 centre (-28.5, -0.369969) radius 4
  circle A15 centre (28.5, -0.369969) radius 4
  circle A16 centre (28.5, -0.369969) radius 1.6
  circle A17 centre (-28.5, -0.369969) radius 1.6
  line L105 (40.5, -0.39984) -> (32.5, -0.39984)
  line L106 (40.5, -4.59984) -> (32.5, -4.59984)
  line L107 (32.5, -0.39984) -> (32.5, -4.59984)
  line L108 (-40.5, -4.59984) -> (-32.5, -4.59984)
  line L109 (-32.5, -4.59984) -> (-32.5, -0.39984)
  line L110 (-40.5, -0.39984) -> (-32.5, -0.39984)
  line L111 (39.5, 3.630031) -> (-39.5, 3.630031)
  point P0 (0, 0)
  point P1 (-28.408002, 50.121275)
  point P2 (28.408002, 50.121275)
  point P3 (-28.408002, -4.369969)
  point P4 (-28.408002, 3.630031)
  point P5 (28.408002, 3.630031)
  point P6 (28.408002, -4.369969)
  point P7 (24.5, -0.369969)
  point P8 (-32.5, -0.369969)
  point P9 (-24.5, -0.369969)
  point P10 (-28.5, -4.369969)
  point P11 (28.408002, -4.368911)
  point P12 (28.408002, 3.628972)
  point P13 (28.408002, 5.130031)
  point P14 (28.5, -4.369969)
  point P15 (32.5, 5.130031)
  dimension "d12" = 3.2
  dimension "d13" = 3.2
  dimension "d44" = 8
  dimension "d45" = 3.2
  dimension "d46" = 3.2
  constraints: 52 end point, 12 horizontal, 8 perpendicular, 7 parallel, 7 point on line, 4 centre point, 4 coincident, 4 collinear, 3 vertical, 18 other
  measures "d12" diameter of A2
  measures "d13" diameter of A3
  measures "d44" distance between parallel lines of L10 L31
  measures "d45" diameter of A16
  measures "d46" diameter of A17
extrude "Выдавливание4" add sketch "Эскиз4" against normal blind 1.5 contours L1 L45 L2 L0 | L22 L23 L24 L1 | L1 L3 L2 L45 | L6 L41 L4 L5 | L6 L7 L4 L41 | L4 L26 L27 L28 | A0 | A1
fillet "Сопряжение2" radius 3 4 edges at (28.408, 64.9623, 7.75) (39.5, 65.2008, 7.75) (-39.5, 65.2008, 7.75) (-28.408, 64.9623, 7.75)
ref_plane "РабПлоскость2" through (-43.5, -51.925, 5) normal (0, 0, 1) x (1, 0, 0)
sketch "Эскиз11" plane through (-39.5, 6.130031, 2) normal (-1, 0, 0) x (0, 0, 1)
  line L0 (-4, 40.944969) -> (-2, 40.944969)
  line L1 (-4, -2) -> (-4, 40.944969)
  line L2 (-4, -2) -> (-2, -2)
  line L3 (-2, 40.944969) -> (-2, -2)
  line L4 (-2, 40.944969) -> (-2, 37.944969)
  line L5 (-2, 37.944969) -> (-1, 36.944969)
  line L6 (-1, 43.365408) -> (-1, -1.5)
  line L7 (-2, 40.944969) -> (-2, 41.344969)
  line L8 (-2, 41.344969) -> (-4.4, 41.344969)
  line L9 (-4.4, 41.344969) -> (-4.4, 37.944969)
  line L10 (-4.4, 37.944969) -> (-4, 37.944969)
  line L11 (-4.4, 37.944969) -> (-6, 36.344969)
  line L12 (-6, 36.344969) -> (-6, 44.365408)
  line L13 (0, 44.365408) -> (5, 44.365408)
  line L14 (-6, 44.365408) -> (0, 44.365408)
  arc A0 (0, 44.365408) -> (-1, 43.365408) centre (0, 43.365408) ccw
  line L15 (-6, 39.894969) -> (-6, 3.254969)
  arc A1 (0.184051, 44.665408) -> (-1.138825, 44.165408) centre (0.184051, 42.665408) ccw
  arc A2 (-1.548, 43.886321) -> (-1.138825, 44.165408) centre (-2.461701, 45.665408) ccw
  arc A3 (-2.461701, 43.665408) -> (-1.548, 43.886321) centre (-2.461701, 45.665408) ccw
  line L16 (-5.89535, 43.665408) -> (6.452, 43.665408)
  arc A4 (0.184051, 44.3892) -> (-0.95613, 43.958252) centre (0.184051, 42.665408) ccw
  arc A5 (-1.421814, 43.640621) -> (-0.95613, 43.958252) centre (-2.461701, 45.665408) ccw
  arc A6 (-2.461701, 43.3892) -> (-1.421814, 43.640621) centre (-2.461701, 45.665408) ccw
  line L17 (-2.461701, 43.3892) -> (-6, 43.3892)
  point P0 (-2, -6.130031)
  point P1 (-1, -6.5)
  point P2 (-0.254287, 44.332537)
  point P3 (-0.101359, 44.365408)
  point P4 (6.5, 44.365408)
  dimension "d61" = 3
  dimension "d62" = 45
  dimension "d63" = 0.4
  dimension "d64" = 0.4
  dimension "d65" = 45
  constraints: 20 end point, 6 point on circle, 5 point on line, 4 perpendicular, 3 centre point, 2 collinear, 2 vertical, 1 tangent, 2 other
  measures "d61" distance of L0.end L4.end
  measures "d62" angle of L6 L5
  measures "d63" distance of L0.end L7.end
  measures "d64" distance of L9.end L10.end
  measures "d65" angle of L11 L9
extrude "Выдавливание11" add sketch "Эскиз11" against normal up to surface (11.091998 mm away) contours L7 L8 L9 L11 L12 L17 A6 A5 L16 A0 L6 L5 L3 | L16 A5 A4 A0 | A4 L14 A0
fillet "Сопряжение9" radius 2 4 edges at (-33.954, 43.075, 1) (-33.954, 44.075, 0) (-33.954, 44.075, -2.4) (-33.954, 49.5192, -4)
fillet "Сопряжение10" radius 0.5 1 edges at (-33.954, 42.475, -4)
fillet "Сопряжение11" radius 0.5 2 edges at (-33.954, 47.475, -2.4) (-33.954, 47.475, 0)
mirror "Зеркальное отражение1" about plane through (0, 0, 0) normal (1, 0, 0) of "Выдавливание11", "Сопряжение9", "Сопряжение10", "Сопряжение11"
fillet "Сопряжение12" radius 1 5 edges at (-28.408, 44.6608, 1) (28.408, 42.6608, 1) (28.408, 45.075, 1) (-28.408, 47.075, 1.5) (28.408, 47.075, 1.5)
